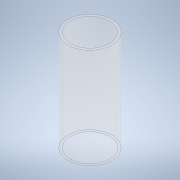
# Autodesk Inventor part: Wash_Chamber_Pipe
Saved by Autodesk Inventor 2022 (Build 260153000, 153)
## iProperties
Created: 2021-10-22
Part Number: Wash_Chamber_Pipe
Material: Plastic, Transparent
Document SubType Name: Modeling
Designer: tgr41
Density: 1.188 g/cm^3
Appearance: Transparent - Clear
Author: tgr41
Autodesk Inventor part; units mm, degrees
ref_plane "YZ Plane" through (0, 0, 0) normal (1, 0, 0) x (0, 1, 0)
ref_plane "XZ Plane" through (0, 0, 0) normal (0, 1, 0) x (-1, 0, 0)
ref_plane "XY Plane" through (0, 0, 0) normal (0, 0, 1) x (1, 0, 0)
sketch "Sketch1" plane through (0, 0, 0) normal (0, 1, 0) x (-1, 0, 0)
  circle A0 centre (0, 0) radius 50.8
  circle A1 centre (0, 0) radius 57.15
  dimension "d0" = 101.6
  dimension "d1" = 114.3
  constraints: 2 centre point, 2 coincident
  measures "d0" diameter of A0
  measures "d1" diameter of A1
extrude "Extrusion1" add sketch "Sketch1" along normal blind 259.334
body "Solid1"
